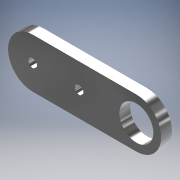
# Autodesk Inventor part: Protection Plates
Saved by Autodesk Inventor 2019.4 (Build 234330000, 330)
## iProperties
Created: 2020-02-04
Part Number: Protection Plates
Material: Aluminum 6061
Document SubType Name: Modeling
Designer: Mark
Mass: 41.5913 g
Surface Area: 66.2862 cm^2
Volume: 15.4042 cm^3
Density: 2.7 g/cm^3
Appearance: Aluminum - Flat
Author: Mark
Autodesk Inventor part; units mm, degrees
ref_plane "YZ Plane" through (0, 0, 0) normal (1, 0, 0) x (0, 1, 0)
ref_plane "XZ Plane" through (0, 0, 0) normal (0, 1, 0) x (-1, 0, 0)
ref_plane "XY Plane" through (0, 0, 0) normal (0, 0, 1) x (1, 0, 0)
sketch "Sketch1" plane through (0, 0, 0) normal (0, 0, 1) x (1, 0, 0)
  circle A0 centre (0, 0) radius 11
  circle A1 centre (-37, 0) radius 2.75
  circle A2 centre (-67, 0) radius 2.75
  line L0 (0, 0) -> (-11, 0) construction
  line L1 (0, 0) -> (11, 0) construction
  line L2 (0, 0) -> (-67, 0) construction
  line L3 (0, -16) -> (-67, -16)
  line L4 (-67, 16) -> (0, 16)
  arc A3 (0, -16) -> (0, 16) centre (0, 0) ccw
  arc A4 (-67, 16) -> (-67, -16) centre (-67, 0) ccw
  point P0 (-33.5, 0)
  dimension "d0" = 22
  dimension "d2" = 5.5
  dimension "d3" = 37
  dimension "d4" = 5.5
  dimension "d5" = 67
  dimension "d6" = 180
  dimension "d7" = 32
  constraints: 12 end point, 4 centre point, 4 point on circle, 4 tangent, 2 collinear, 2 point on line, 1 coincident, 1 horizontal, 1 horizontal alignment, 1 midpoint, 1 parallel, 2 other
  measures "d2" diameter of A1
  measures "d3" distance of L0.start A1.centre
  measures "d4" diameter of A2
  measures "d5" distance of L0.start L2.end
  measures "d6" angle of L0 L1
  measures "d7" distance between parallel lines of L3 L4
extrude "Extrusion1" add sketch "Sketch1" along normal blind 7
body "Solid1"
